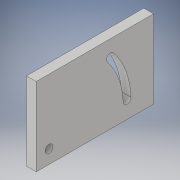
# Autodesk Inventor part: third odomitry wheel
Saved by Autodesk Inventor 2019 (Build 230136000, 136)
## iProperties
Created: 2020-10-13
Part Number: third odomitry wheel
Material: Generic
Document SubType Name: Modeling
Designer: User
Density: 1 g/cm^3
Appearance: Default
Author: User
Autodesk Inventor part; units mm, degrees
ref_plane "YZ Plane" through (0, 0, 0) normal (1, 0, 0) x (0, 1, 0)
ref_plane "XZ Plane" through (0, 0, 0) normal (0, 1, 0) x (-1, 0, 0)
ref_plane "XY Plane" through (0, 0, 0) normal (0, 0, 1) x (1, 0, 0)
sketch "Sketch1" plane through (0, 0, 0) normal (1, 0, 0) x (0, 1, 0)
  line L0 (0, 0) -> (50.8, 0)
  line L1 (50.8, 0) -> (50.8, -76.2)
  line L2 (50.8, -76.2) -> (0, -76.2)
  line L3 (0, -76.2) -> (0, 0)
  dimension "d0" = 76.2
  dimension "d1" = 50.8
  constraints: 8 end point, 2 parallel, 1 horizontal, 1 perpendicular
  measures "d0" distance of L0.end L1.end
  measures "d1" distance of L1.end L2.end
extrude "Extrusion1" add sketch "Sketch1" along normal blind 6.35
sketch "Sketch2" plane through (6.35, 0, 0) normal (1, 0, 0) x (0, 0, -1)
  circle A0 centre (8.2479, 8.89) radius 2.54
  line L0 (0, 0) -> (76.2, 0) projected
  arc A1 (59.001, 11.0708) -> (48.1249, 40.3615) centre (8.2479, 8.89) ccw construction
  arc A2 (61.5387, 11.1798) -> (50.1188, 41.9351) centre (8.2479, 8.89) ccw
  arc A3 (56.4634, 10.9617) -> (46.1311, 38.788) centre (8.2479, 8.89) ccw
  arc A4 (56.4634, 10.9617) -> (61.5387, 11.1798) centre (59.001, 11.0708) ccw
  arc A5 (50.1188, 41.9351) -> (46.1311, 38.788) centre (48.1249, 40.3615) ccw
  dimension "d4" = 8.89
  dimension "d5" = 50.8
  dimension "d6" = 5.08
  dimension "d7" = 5.08
  constraints: 10 point on circle, 6 centre point, 4 tangent, 1 coincident
  measures "d4" distance from line of L0 A0.centre
  measures "d5" radius of A1
  measures "d6" diameter of A4
  measures "d7" diameter of A0
extrude "Extrusion2" cut sketch "Sketch2" against normal through all
sketch "Sketch3" plane through (0, 0, -76.2) normal (0, -1, 0) x (1, 0, 0)
  line L0 (0, 0) -> (0, 76.2) projected
  line L1 (0, 0) -> (6.35, 0) projected
  line L2 (6.35, 76.2) -> (6.35, 0) projected
  line L3 (0, 76.2) -> (6.35, 76.2) projected
  point P0 (3.6586, 56.6207)
  point P1 (3.9004, 5.8386)
hole "Hole1" at (3.6586, 0, -19.5793) at (3.9004, 0, -70.3614) direction (0, 1, 0) diameter 1.9304 depth 7.6708 tip angle 118
body "Solid1"
